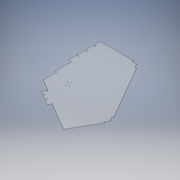
# Autodesk Inventor part: Acrylic_bottom_camera
Saved by Autodesk Inventor 2019.4 (Build 234330000, 330)
## iProperties
Created: 2020-02-04
Part Number: Acrylic_bottom_camera
Material: Generic
Document SubType Name: Modeling
Designer: Jorian Brusind
Density: 1 g/cm^3
Appearance: Polycarbonate - Clear
Author: Jorian Brusind
Autodesk Inventor part; units mm, degrees
ref_plane "YZ Plane" through (0, 0, 0) normal (1, 0, 0) x (0, 1, 0)
ref_plane "XZ Plane" through (0, 0, 0) normal (0, 1, 0) x (-1, 0, 0)
ref_plane "XY Plane" through (0, 0, 0) normal (0, 0, 1) x (1, 0, 0)
sketch "Sketch1" plane through (0, 0, 0) normal (0, 1, 0) x (-1, 0, 0)
  line L0 (349.8743, 0) -> (258.4057, -158.4282)
  line L1 (174.9371, -303) -> (-174.9371, -303)
  line L2 (-174.9371, -303) -> (-349.8743, 0)
  line L3 (-349.8743, 0) -> (-174.9371, 303)
  line L4 (-174.9371, 303) -> (174.9371, 303)
  line L5 (258.4057, 158.4282) -> (349.8743, 0)
  line L6 (0, 0) -> (-8, 0)
  line L7 (-8, 0) -> (-8, -303)
  line L8 (-8, -303) -> (8, -303)
  line L9 (8, -303) -> (8, 0)
  line L10 (8, 0) -> (-8, 0)
  circle A0 centre (0, 0) radius 2.5
  line L11 (258.4057, 158.4282) -> (-4, 6.9282)
  line L12 (4, -6.9282) -> (266.4057, 144.5718)
  line L13 (-4, 6.9282) -> (4, -6.9282)
  line L14 (-266.4057, 144.5718) -> (-4, -6.9282)
  line L15 (4, 6.9282) -> (-258.4057, 158.4282)
  line L16 (-4, -6.9282) -> (4, 6.9282)
  line L17 (8, -4.6188) -> (8, -151.5)
  line L18 (8, -151.5) -> (-8, -151.5)
  line L19 (-8, -151.5) -> (-8, -303)
  line L20 (-8, -4.6188) -> (-4, -6.9282)
  line L21 (4, -6.9282) -> (-4, -6.9282)
  line L22 (-266.4057, 144.5718) -> (-258.4057, 158.4282)
  line L23 (-127.2028, 82.6782) -> (-135.2028, 68.8218)
  line L24 (-135.2028, 68.8218) -> (-8, -4.6188)
  line L25 (-266.4057, 144.5718) -> (-349.8743, 0)
  line L26 (-174.9371, -303) -> (-349.8743, 0)
  line L27 (-174.9371, -303) -> (-8, -303)
  line L28 (0, 9.2376) -> (8, 0)
  dimension "d0" = 303
  dimension "d1" = 303
  dimension "d2" = 8
  dimension "d3" = 16
  dimension "d4" = 5
  dimension "d7" = 360
  constraints: 58 end point, 7 point on line, 5 collinear, 4 midpoint, 4 perpendicular, 2 coincident, 2 parallel, 1 centre point, 1 horizontal, 35 other
  measures "d0" distance from line of point (0, 0) L1
  measures "d1" vertical distance of L4.end L0.start
  measures "d2" distance of L6.start L6.end
  measures "d3" distance of L8.end L7.end
  measures "d4" diameter of A0
extrude "Extrusion1" add sketch "Sketch1" along normal blind 3 contours L1 L7 L18 L9 | L1 L2 L3 L14 L7 | L18 L7 L14 L21 L12 L9 | L12 L13 A0 L10 L9 | L14 L23 L15 L11 L13 A0 L6 L7 | L7 L6 A0 L16 L14 | L10 A0 L16 L28 | L21 L16 A0 L13 | L3 L15 L23 L14 | A0 L13 L10 | L10 L16 A0 | L28 L15 L16 | L16 A0 L13 L11 L28 | A0 L16 L13 | A0 L13 L6 | L6 L16 A0 | L13 A0 L16
sketch "Sketch2" plane through (0, 3, 0) normal (0, 1, 0) x (1, 0, 0)
  line L0 (-8, 303) -> (-8, 0) projected
  line L1 (-8, 0) -> (-8, 151.5)
  line L2 (-8, 151.5) -> (8, 151.5)
  line L3 (8, 151.5) -> (8, 0)
  line L4 (8, 0) -> (-8, 0)
  line L5 (0, -9.2376) -> (258.4057, -158.4282) projected
  line L6 (258.4057, -158.4282) -> (126.3368, -82.1782)
  line L7 (126.3368, -82.1782) -> (134.8368, -67.4558)
  line L8 (134.8368, -67.4558) -> (266.9057, -143.7058)
  line L9 (266.9057, -143.7058) -> (258.4057, -158.4282)
  point P0 (0, 0)
  dimension "d11" = 151.5
  dimension "d12" = 16
  dimension "d13" = 152.5
  dimension "d14" = 17
  constraints: 16 end point, 4 parallel, 2 perpendicular, 1 midpoint, 1 point on line
  measures "d11" distance of L0.end L1.end
  measures "d12" distance of L1.end L2.end
  measures "d13" distance of L5.end L6.end
  measures "d14" distance of L6.end L7.end
extrude "Extrusion2" cut sketch "Sketch2" against normal blind 3
sketch "Sketch3" plane through (0, 3, 0) normal (0, 1, 0) x (1, 0, 0)
  line L0 (174.9371, 303) -> (-8, 303) projected
  line L1 (174.9371, 303) -> (149.9371, 303)
  line L2 (149.9371, 303) -> (149.9371, 297)
  line L3 (149.9371, 297) -> (174.9371, 297)
  line L4 (174.9371, 297) -> (174.9371, 303)
  line L5 (349.8743, 0) -> (174.9371, 303) projected
  line L6 (174.9371, 303) -> (187.4371, 281.3494)
  line L7 (187.4371, 281.3494) -> (182.241, 278.3494)
  line L8 (182.241, 278.3494) -> (169.741, 300)
  line L9 (169.741, 300) -> (174.9371, 303)
  line L10 (349.8743, 0) -> (337.3743, 21.6506)
  line L11 (337.3743, 21.6506) -> (332.1781, 18.6506)
  line L12 (332.1781, 18.6506) -> (344.6781, -3)
  line L13 (344.6781, -3) -> (349.8743, 0)
  line L14 (349.8743, 0) -> (337.3743, -21.6506)
  line L15 (337.3743, -21.6506) -> (332.1781, -18.6506)
  line L16 (332.1781, -18.6506) -> (344.6781, 3)
  line L17 (344.6781, 3) -> (349.8743, 0)
  line L18 (349.8743, 0) -> (266.9057, -143.7058) projected
  line L19 (349.8743, 0) -> (374.8743, 0) construction
  point P0 (0, 0)
  dimension "d17" = 25
  dimension "d18" = 6
  dimension "d19" = 25
  dimension "d20" = 6
  dimension "d21" = 25
  dimension "d22" = 6
  dimension "d23" = 25
  dimension "d24" = 120
  dimension "d25" = 6
  constraints: 34 end point, 8 parallel, 4 perpendicular, 3 point on line, 1 collinear, 1 equal length, 1 horizontal
  measures "d17" distance of L0.start L1.end
  measures "d18" distance of L2.end L1.end
  measures "d19" distance of L0.start L6.end
  measures "d20" distance of L6.end L7.end
  measures "d21" distance of L5.start L10.end
  measures "d22" distance of L11.end L10.end
  measures "d23" distance of L5.start L14.end
  measures "d24" angle of L14 L19
  measures "d25" distance of L14.end L15.end
extrude "Extrusion3" cut sketch "Sketch3" against normal blind 3
sketch "Sketch4" plane through (0, 3, 0) normal (0, 1, 0) x (1, 0, 0)
  line L0 (-55.0368, 49.6734) -> (70.5368, -22.8266)
  line L1 (70.5368, -22.8266) -> (55.0368, -49.6734)
  line L2 (55.0368, -49.6734) -> (-70.5368, 22.8266)
  line L3 (-70.5368, 22.8266) -> (-55.0368, 49.6734)
  line L4 (-55.0368, 49.6734) -> (55.0368, -49.6734) construction
  line L5 (70.5368, -22.8266) -> (-70.5368, 22.8266) construction
  line L6 (-55.0368, 49.6734) -> (89.9632, 49.6734) construction
  line L7 (-15.5, -72.5) -> (-15.5, 72.5)
  line L8 (-15.5, 72.5) -> (15.5, 72.5)
  line L9 (15.5, 72.5) -> (15.5, -72.5)
  line L10 (15.5, -72.5) -> (-15.5, -72.5)
  line L11 (-15.5, -72.5) -> (15.5, 72.5) construction
  line L12 (-15.5, 72.5) -> (15.5, -72.5) construction
  line L13 (-8, 0) -> (8, 0) projected
  line L14 (-15.5, -72.5) -> (129.5, -72.5) construction
  point P0 (0, 0)
  dimension "d28" = 145
  dimension "d29" = 30
  dimension "d30" = 31
  dimension "d31" = 145
  dimension "d32" = 90
  dimension "d33" = 31
  constraints: 28 end point, 4 midpoint, 4 parallel, 3 perpendicular, 2 equal length, 2 horizontal
  measures "d28" distance of L0.start L0.end
  measures "d29" angle of L0 L6
  measures "d30" distance of L0.end L1.end
  measures "d31" distance of L7.start L7.end
  measures "d32" angle of L14 L7
  measures "d33" distance of L7.end L8.end
extrude "Extrusion4" cut sketch "Sketch4" against normal blind 3
sketch "Sketch5" plane through (0, 3, 0) normal (0, 1, 0) x (1, 0, 0)
  line L0 (-1, 151.5) -> (-1, 191.5)
  circle A0 centre (-1, 191.5) radius 2.75
  circle A1 centre (-1, 231.5) radius 2.75
  circle A2 centre (-1, 271.5) radius 2.75
  circle A3 centre (0, 0) radius 0.5
  line L1 (126.3368, -82.1782) -> (134.8368, -67.4558) projected
  line L2 (126.3368, -82.1782) -> (129.3368, -76.9821)
  line L3 (129.3368, -76.9821) -> (103.3561, -61.9821)
  line L4 (103.3561, -61.9821) -> (77.3753, -46.9821)
  circle A4 centre (103.3561, -61.9821) radius 2.75
  circle A5 centre (77.3753, -46.9821) radius 2.75
  line L5 (-8, 303) -> (-8, 151.5) projected
  dimension "d36" = 40
  dimension "d37" = 5.5
  dimension "d40" = 40
  dimension "d45" = 1
  dimension "d46" = 6
  dimension "d47" = 30
  dimension "d48" = 30
  dimension "d49" = 5.5
  dimension "d50" = 5.5
  dimension "d53" = 7
  constraints: 8 end point, 6 centre point, 4 coincident, 2 point on line, 2 vertical, 1 perpendicular, 4 other
  measures "d36" distance of L0.start L0.end
  measures "d37" diameter of A0
  measures "d40" distance of A0.centre A1.centre
  measures "d45" diameter of A3
  measures "d46" distance of L1.start L2.end
  measures "d47" distance of L2.end L3.end
  measures "d48" distance of L3.end L4.end
  measures "d49" diameter of A4
  measures "d50" diameter of A5
  measures "d53" distance between parallel lines of L5 L0
extrude "Extrusion5" cut sketch "Sketch5" against normal blind 3 contours A0 | A1 | A2 | A4 L4 L3 | A5 | L3 L4 A4
sketch "Sketch6" plane through (0, 3, 0) normal (0, 1, 0) x (1, 0, 0)
  line L0 (-8, 303) -> (-8, 151.5) projected
  line L1 (-8, 303) -> (344, 303)
  line L2 (344, 303) -> (344, -147)
  line L3 (344, -147) -> (-8, -147)
  line L4 (-8, -147) -> (-8, 303)
  point P0 (0, 0)
  dimension "d54" = 352
  dimension "d55" = 450
  constraints: 8 end point, 2 parallel, 1 horizontal, 1 perpendicular
  measures "d54" distance of L2.end L3.end
  measures "d55" distance of L1.end L2.end
sketch "Sketch7" plane through (0, 3, 0) normal (0, 1, 0) x (1, 0, 0)
  line L0 (0, 0) -> (86.6025, 50)
  line L1 (0, 0) -> (100, 0) construction
  line L2 (86.6025, 50) -> (91.8525, 40.9067)
  circle A0 centre (91.8525, 40.9067) radius 1.1
  line L3 (86.6025, 50) -> (89.2006, 51.5)
  line L4 (86.6025, 50) -> (89.6025, 50) construction
  circle A1 centre (81.3525, 59.0933) radius 1.1
  circle A2 centre (102.6779, 47.1567) radius 1.1
  circle A3 centre (92.1779, 65.3433) radius 1.1
  dimension "d56" = 100
  dimension "d57" = 30
  dimension "d58" = 10.5
  dimension "d59" = 90
  dimension "d60" = 2.2
  dimension "d61" = 3
  dimension "d62" = 30
  dimension "d65" = 21
  dimension "d68" = 12.5
  constraints: 10 end point, 4 centre point, 2 equal length, 2 horizontal, 1 coincident, 8 other
  measures "d56" distance of L0.start L0.end
  measures "d57" angle of L1 L0
  measures "d58" distance of L0.end L2.end
  measures "d59" angle of L0 L2
  measures "d60" diameter of A0
  measures "d61" distance of L0.end L3.end
  measures "d62" angle of L4 L3
  measures "d65" distance of A0.centre A1.centre
  measures "d68" distance of A0.centre A2.centre
extrude "Extrusion6" cut sketch "Sketch7" against normal blind 5
body "Solid1"
